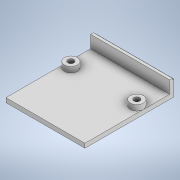
# Autodesk Inventor part: ExpansionCard_SelfTapping_Lid
Saved by Autodesk Inventor 2022 (Build 260153000, 153)
## iProperties
Created: 2022-05-23
Part Number: ExpansionCard_SelfTapping_Lid
Material: Generic
Document SubType Name: Modeling
Designer: SHOP-Station5
Density: 1 g/cm^3
Appearance: Default
Author: SHOP-Station5
Autodesk Inventor part; units mm, degrees
ref_plane "YZ Plane" through (0, 0, 0) normal (1, 0, 0) x (0, 1, 0)
ref_plane "XZ Plane" through (0, 0, 0) normal (0, 1, 0) x (-1, 0, 0)
ref_plane "XY Plane" through (0, 0, 0) normal (0, 0, 1) x (1, 0, 0)
sketch "Sketch1" plane through (0, 0, 0) normal (0, 1, 0) x (-1, 0, 0)
  line L0 (-27.0524, -30.5) -> (0, -30.5)
  line L1 (-27.0524, -30.5) -> (-27.0524, 0)
  line L2 (-27.0524, 0) -> (0, 0)
  line L3 (0, 0) -> (0, -30.5)
  point P0 (-13.5262, -30.5)
  constraints: 8 end point, 1 vertical
extrude "Extrusion1" add sketch "Sketch1" along normal blind 1.5
sketch "Sketch2" plane through (0, 0, 0) normal (0, -1, 0) x (1, 0, 0)
  circle A0 centre (2.2262, -20) radius 2.2262
  circle A1 centre (24.8262, -20) radius 2.2262
  point P0 (0, 0)
  point P1 (13.5262, -30.5)
  point P2 (27.0524, -30.5)
  constraints: 2 centre point
extrude "Extrusion2" add sketch "Sketch2" against normal blind 3.4
sketch "Sketch3" plane through (0, 0, 0) normal (0, -1, 0) x (1, 0, 0)
  circle A0 centre (24.8262, -19.9938) radius 1.016
  circle A1 centre (2.2262, -20) radius 1.016
  point P0 (0, 0)
  point P1 (13.5262, 0)
  point P2 (1.4262, -20)
  point P3 (0, -30.5)
  dimension "d4" = 2.032
  constraints: 2 centre point
  measures "d4" diameter of A0
extrude "Extrusion3" cut sketch "Sketch3" against normal up to surface (3.4 mm away)
sketch "Sketch4" plane through (0, 0, 0) normal (0, -1, 0) x (1, 0, 0)
  circle A0 centre (24.8262, -19.9938) radius 2.032
  circle A1 centre (2.2262, -20) radius 2.032
  line L0 (2.2262, -20) -> (0, -20)
  line L1 (0, -20) -> (0, -30.5)
  line L2 (0, -30.5) -> (0, 0) projected
  point P0 (13.5262, 0)
  dimension "d7" = 4.064
  dimension "d8" = 4.064
  constraints: 4 end point, 2 centre point, 1 coincident, 1 horizontal
  measures "d7" diameter of A0
  measures "d8" diameter of A1
extrude "Extrusion4" cut sketch "Sketch4" against normal blind 2.051
sketch "Sketch5" plane through (27.0524, 0, -30.5) normal (0, 0, -1) x (-1, 0, 0)
  line L0 (27.0524, 1.5) -> (27.0524, 3.4) projected
  line L1 (27.0524, 1.5) -> (27.0524, 5.3)
  line L2 (27.0524, 5.3) -> (0, 5.3)
  line L3 (0, 1.5) -> (0, 3.4) projected
  line L4 (0, 5.3) -> (0, 1.5)
  line L5 (0, 1.5) -> (27.0524, 1.5) projected
  line L6 (27.0524, 1.5) -> (0, 1.5)
  point P0 (27.0524, 0)
  dimension "d11" = 3.8
  constraints: 8 end point, 2 perpendicular, 2 point on line, 1 collinear
  measures "d11" distance of L1.start L1.end
extrude "Extrusion5" add sketch "Sketch5" against normal blind 1.5
sketch "Sketch6" plane through (0, 5.3, -30.5) normal (0, 1, 0) x (1, 0, 0)
  line L0 (27.0524, -10.5) -> (27.0524, -1.5) projected
  line L1 (27.0524, -1.5) -> (27.0524, -0.55)
  line L2 (27.0524, 0) -> (27.0524, -1.5) projected
  line L3 (27.0524, -0.55) -> (0, -0.55)
  line L4 (27.0524, 0) -> (0, 0) projected
  line L5 (0, -0.55) -> (0, -1.5)
  line L6 (0, 0) -> (0, -30.5) projected
  line L7 (27.0524, -1.5) -> (0, -1.5) projected
  line L8 (27.0524, -1.5) -> (0, -1.5)
  dimension "d21" = 0.95
  constraints: 8 end point, 1 collinear, 1 horizontal, 1 parallel, 1 point on line
  measures "d21" distance of L0.end L1.end
extrude "Extrusion6" add sketch "Sketch6" along normal blind 0.5 contours L7 L5 L3 L1
body "Solid1"
